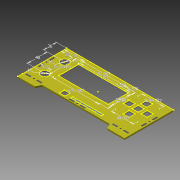
# Autodesk Inventor part: Front Panel
Saved by Autodesk Inventor 2014 (Build 180170000, 170)
## iProperties
Created: 2013-07-14
Part Number: Front Panel
Material: Generic
Document SubType Name: Modeling
Designer: james
Density: 1 g/cm^3
Appearance: Default
Author: james
Autodesk Inventor part; units mm, degrees
ref_plane "YZ Plane" through (0, 0, 0) normal (1, 0, 0) x (0, 1, 0)
ref_plane "XZ Plane" through (0, 0, 0) normal (0, 1, 0) x (-1, 0, 0)
ref_plane "XY Plane" through (0, 0, 0) normal (0, 0, 1) x (1, 0, 0)
sketch "Sketch1" plane through (0, 0, 0) normal (0, 0, 1) x (1, 0, 0)
  line L0 (-107.95, 44.45) -> (107.95, 44.45)
  line L1 (-107.95, -54.45) -> (-72.95, -54.45)
  line L2 (-72.95, -54.45) -> (-67.95, -44.45)
  line L3 (67.95, -44.45) -> (-67.95, -44.45)
  line L4 (107.95, -54.45) -> (72.95, -54.45)
  line L5 (72.95, -54.45) -> (67.95, -44.45)
  line L6 (-107.95, 44.45) -> (-107.95, -54.45)
  line L7 (107.95, 44.45) -> (107.95, -54.45)
  point P0 (0, 0)
  dimension "d36" = 88.9
  dimension "d38" = 215.9
  dimension "d39" = 44.45
  dimension "d40" = 107.95
  dimension "d41" = 98.9
  dimension "d42" = 10
  dimension "d43" = 116.565
  dimension "d44" = 35
  dimension "d45" = 35
  dimension "d46" = 116.565
  dimension "d47" = 40
  constraints: 16 end point, 2 parallel, 1 horizontal, 1 perpendicular
  measures "d36" distance between parallel lines of L3 L0
  measures "d38" distance of L0.start L0.end
  measures "d39" distance from line of point (0, 0) L0
  measures "d40" distance from line of point (0, 0) L6
  measures "d41" distance of L0.start L1.start
  measures "d42" distance between parallel lines of L1 L3
  measures "d43" angle of L1 L2
  measures "d44" distance of L4.start L4.end
  measures "d45" distance of L1.start L1.end
  measures "d46" angle of L4 L5
  measures "d47" distance from line of L7 L3.start
extrude "Face ext" add sketch "Sketch1" along normal blind 3
sketch "Cutouts - skt" plane through (0, 0, 3) normal (0, 0, 1) x (1, 0, 0)
  line L0 (107.95, 44.45) -> (-107.95, 44.45) projected
  line L1 (63.8676, -13.289) -> (63.8676, -1.2663)
  line L2 (75.89, -13.289) -> (63.8676, -13.289)
  line L3 (75.89, -1.2663) -> (75.89, -13.289)
  line L4 (63.8676, -1.2663) -> (75.89, -1.2663)
  line L5 (46.0028, 16.7255) -> (58.0255, 16.7255)
  line L6 (46.0028, 4.7026) -> (46.0028, 16.7255)
  line L7 (58.0255, 4.7026) -> (46.0028, 4.7026)
  line L8 (58.0255, 16.7255) -> (58.0255, 4.7026)
  line L9 (75.9748, 33.8704) -> (75.9748, 21.8478)
  line L10 (63.9944, 33.8704) -> (75.9748, 33.8704)
  line L11 (63.9944, 21.8478) -> (63.9944, 33.8704)
  line L12 (75.9748, 21.8478) -> (63.9944, 21.8478)
  line L13 (63.9521, 16.7677) -> (75.9324, 16.7677)
  line L14 (63.9521, 4.7874) -> (63.9521, 16.7677)
  line L15 (75.9324, 4.7874) -> (63.9521, 4.7874)
  line L16 (75.9324, 16.7677) -> (75.9324, 4.7874)
  line L17 (94.0088, 4.8721) -> (94.0088, 16.8525)
  line L18 (82.0285, 4.8721) -> (94.0088, 4.8721)
  line L19 (82.0285, 16.8525) -> (82.0285, 4.8721)
  line L20 (94.0088, 16.8525) -> (82.0285, 16.8525)
  line L21 (27.7989, -11.6866) -> (-67.95, -11.6866)
  line L22 (-67.95, 28.3134) -> (25.7989, 28.3134)
  line L23 (32.0499, 28.3134) -> (32.0499, -11.6866)
  circle A0 centre (-85.95, 18.45) radius 8
  circle A1 centre (-85.95, -21.55) radius 8
  line L24 (-67.95, 28.3134) -> (32.0499, 28.3134)
  line L25 (32.0499, 28.3134) -> (32.0499, -11.6866)
  line L26 (32.0499, -11.6866) -> (-67.95, -11.6866)
  line L27 (-67.95, -11.6866) -> (-67.95, 28.3134)
  line L28 (63.9944, 33.8704) -> (75.9748, 33.8704)
  line L29 (75.9748, 33.8704) -> (75.9748, 21.8478)
  line L30 (75.9748, 21.8478) -> (63.9944, 21.8478)
  line L31 (63.9944, 21.8478) -> (63.9944, 33.8704)
  line L32 (82.0285, 16.8525) -> (94.0088, 16.8525)
  line L33 (94.0088, 16.8525) -> (94.0088, 4.8721)
  line L34 (94.0088, 4.8721) -> (82.0285, 4.8721)
  line L35 (82.0285, 4.8721) -> (82.0285, 16.8525)
  line L36 (63.9521, 16.7677) -> (75.9324, 16.7677)
  line L37 (75.9324, 16.7677) -> (75.9324, 4.7874)
  line L38 (75.9324, 4.7874) -> (63.9521, 4.7874)
  line L39 (63.9521, 4.7874) -> (63.9521, 16.7677)
  line L40 (46.0028, 16.7255) -> (58.0255, 16.7255)
  line L41 (58.0255, 16.7255) -> (58.0255, 4.7026)
  line L42 (58.0255, 4.7026) -> (46.0028, 4.7026)
  line L43 (46.0028, 4.7026) -> (46.0028, 16.7255)
  line L44 (63.8676, -1.2663) -> (75.89, -1.2663)
  line L45 (75.89, -1.2663) -> (75.89, -13.289)
  line L46 (75.89, -13.289) -> (63.8676, -13.289)
  line L47 (63.8676, -13.289) -> (63.8676, -1.2663)
  line L48 (-36.7815, -30.9654) -> (-26.011, -30.9654)
  line L49 (-26.011, -30.9654) -> (-26.011, -40.9281)
  line L50 (-26.011, -40.9281) -> (-36.7815, -40.9281)
  line L51 (-36.7815, -40.9281) -> (-36.7815, -30.9654)
  line L52 (-16.5867, -34.4658) -> (45.1738, -34.4658) construction
  line L53 (45.1738, -34.4658) -> (45.1738, -38.1955) construction
  line L54 (45.1738, -38.1955) -> (-16.5867, -38.1955) construction
  line L55 (-16.5867, -38.1955) -> (-16.5867, -34.4658) construction
  line L56 (-107.95, 44.45) -> (-107.95, -54.45) projected
  point P0 (-107.95, -44.45)
  point P1 (0, 0)
  point P2 (-70.7327, 35.8725)
  point P3 (22.3305, 35.8725)
  point P4 (22.3305, -19.1888)
  point P5 (-70.7327, -19.1888)
  point P6 (48.035, 31.7962)
  point P7 (92.0616, 31.7962)
  point P8 (48.035, -12.2207)
  point P9 (92.0616, -12.2207)
  point P10 (48.035, 31.7962)
  point P11 (92.0616, 31.7962)
  point P12 (92.0616, -12.2207)
  point P13 (48.035, -12.2207)
  point P14 (-70.7327, 35.8725)
  point P15 (22.3305, 35.8725)
  point P16 (22.3305, -19.1888)
  point P17 (-70.7327, -19.1888)
  dimension "d8" = 16
  dimension "d9" = 16
  dimension "d13" = 26
  dimension "d48" = 40
  dimension "d49" = 99.9999
  dimension "d50" = 40
  dimension "d51" = 93.0632
  dimension "d52" = 93.0632
  dimension "d53" = 55.0612
  dimension "d54" = 55.0612
  dimension "d55" = 8.5775
  dimension "d57" = 7.5591
  dimension "d59" = 44.0266
  dimension "d60" = 44.0266
  dimension "d61" = 22
  dimension "d62" = 22
  dimension "d90" = 40
  dimension "d91" = 18
  constraints: 102 end point, 14 parallel, 8 coincident, 7 horizontal, 7 perpendicular, 2 centre point, 2 other
  measures "d8" diameter of A0
  measures "d9" diameter of A1
  measures "d13" distance from line of L0 A0.centre
  measures "d48" distance of A1.centre A0.centre
  measures "d49" distance of L22.start L24.end
  measures "d50" distance of L23.start L23.end
  measures "d51" distance of point (22.331, 35.872) point (-70.733, 35.872)
  measures "d52" distance of point (22.331, -19.189) point (-70.733, -19.189)
  measures "d53" distance of point (22.331, -19.189) point (22.331, 35.872)
  measures "d54" distance of point (-70.733, -19.189) point (-70.733, 35.872)
  measures "d55" distance from line of L0 point (22.331, 35.872)
  measures "d57" distance from line of L22 point (22.331, 35.872)
  measures "d59" distance of point (92.062, -12.221) point (48.035, -12.221)
  measures "d60" distance of point (92.062, 31.796) point (48.035, 31.796)
  measures "d61" distance from line of L56 A0.centre
  measures "d62" distance from line of L56 A1.centre
  measures "d90" distance between parallel lines of L56 L27
  measures "d91" distance from line of L27 A0.centre
sketch3d "3D Sketch1"
extrude "Cut-outs ext" cut sketch "Cutouts - skt" against normal through all
hole "Hole1" at (-70.7327, 35.8725, 3) at (-70.7327, -19.1888, 3) at (22.3305, -19.1888, 3) at (22.3305, 35.8725, 3) at (48.035, -12.2207, 3) at (48.035, 31.7962, 3) at (92.0616, 31.7962, 3) at (92.0616, -12.2207, 3) direction (0, 0, -1) diameter 3 end through all
sketch "Mating Holes" plane through (0, 0, 3) normal (0, 0, 1) x (1, 0, 0)
  line L0 (107.95, 44.45) -> (-107.95, 44.45) projected
  line L1 (-107.95, 44.45) -> (-107.95, -54.45) projected
  line L2 (-67.95, -44.45) -> (67.95, -44.45) projected
  line L3 (107.95, -54.45) -> (107.95, 44.45) projected
  circle A0 centre (-103.95, 0) radius 1.5
  line L4 (-105.5, -6) -> (-102.4, -6)
  line L5 (-102.4, -6) -> (-102.4, -16.1)
  line L6 (-102.4, -16.1) -> (-105.5, -16.1)
  line L7 (-105.5, -16.1) -> (-105.5, -6)
  line L8 (-105.5, 16.0999) -> (-102.4, 16.0999)
  line L9 (-102.4, 16.0999) -> (-102.4, 5.9999)
  line L10 (-102.4, 5.9999) -> (-105.5, 5.9999)
  line L11 (-105.5, 5.9999) -> (-105.5, 16.0999)
  circle A1 centre (103.95, 0) radius 1.5
  line L12 (102.4, -6) -> (105.5, -6)
  line L13 (105.5, -6) -> (105.5, -16.1)
  line L14 (105.5, -16.1) -> (102.4, -16.1)
  line L15 (102.4, -16.1) -> (102.4, -6)
  line L16 (102.4, 16.0999) -> (105.5, 16.0999)
  line L17 (105.5, 16.0999) -> (105.5, 5.9999)
  line L18 (105.5, 5.9999) -> (102.4, 5.9999)
  line L19 (102.4, 5.9999) -> (102.4, 16.0999)
  point P0 (0, 0)
  dimension "d63" = 3
  dimension "d75" = 44.45
  dimension "d79" = 3.1
  dimension "d80" = 10.1
  dimension "d81" = 6
  dimension "d85" = 3.1
  dimension "d86" = 10.1
  dimension "d87" = 5.9999
  dimension "d88" = 1.55
  dimension "d89" = 1.55
  dimension "d92" = 3
  dimension "d93" = 3.1
  dimension "d94" = 10.1
  dimension "d95" = 6
  dimension "d96" = 3.1
  dimension "d97" = 10.1
  dimension "d98" = 5.9999
  dimension "d99" = 1.55
  dimension "d100" = 1.55
  dimension "d101" = 4
  dimension "d102" = 44.45
  dimension "d103" = 4
  dimension "d104" = 88.9
  constraints: 32 end point, 8 parallel, 4 horizontal, 4 perpendicular, 2 centre point
  measures "d63" diameter of A0
  measures "d75" distance from line of L0 A0.centre
  measures "d79" distance of L5.end L6.end
  measures "d80" distance of L4.end L5.end
  measures "d81" vertical distance of L4.end A0.centre
  measures "d85" distance of L9.end L10.end
  measures "d86" distance of L8.end L9.end
  measures "d87" distance from line of L10 A0.centre
  measures "d88" distance from line of A0.centre L9
  measures "d89" distance from line of L5 A0.centre
  measures "d92" diameter of A1
  measures "d93" distance of L14.start L14.end
  measures "d94" distance of L13.start L14.start
  measures "d95" vertical distance of L13.start A1.centre
  measures "d96" distance of L18.start L18.end
  measures "d97" distance of L17.start L18.start
  measures "d98" distance from line of L18 A1.centre
  measures "d99" distance from line of A1.centre L17
  measures "d100" distance from line of L13 A1.centre
  measures "d101" distance from line of L3 A1.centre
  measures "d102" distance from line of L0 A1.centre
  measures "d103" distance from line of L1 A0.centre
  measures "d104" distance between parallel lines of L2 L0
extrude "Side Panel Slots" cut sketch "Mating Holes" against normal through all
sketch "Bottom Panel Slots" plane through (0, 0, 3) normal (0, 0, 1) x (1, 0, 0)
  line L0 (-107.95, 44.45) -> (-107.95, -54.45) projected
  line L1 (-107.95, -54.45) -> (-72.95, -54.45) projected
  line L2 (72.95, -54.45) -> (107.95, -54.45) projected
  circle A0 centre (-87.945, -41.45) radius 1.5
  line L3 (-93.945, -39.9) -> (-104.045, -39.9)
  line L4 (-104.045, -39.9) -> (-104.045, -43)
  line L5 (-104.045, -43) -> (-93.945, -43)
  line L6 (-93.945, -43) -> (-93.945, -39.9)
  line L7 (-81.945, -39.9) -> (-71.845, -39.9)
  line L8 (-71.845, -39.9) -> (-71.845, -43)
  line L9 (-71.845, -43) -> (-81.945, -43)
  line L10 (-81.945, -43) -> (-81.945, -39.9)
  circle A1 centre (87.013, -41.45) radius 1.5
  line L11 (93.013, -42.95) -> (103.113, -42.95)
  line L12 (103.113, -42.95) -> (103.113, -39.85)
  line L13 (103.113, -39.85) -> (93.013, -39.85)
  line L14 (93.013, -39.85) -> (93.013, -42.95)
  line L15 (81.013, -39.85) -> (70.913, -39.85)
  line L16 (70.913, -39.85) -> (70.913, -42.95)
  line L17 (70.913, -42.95) -> (81.013, -42.95)
  line L18 (81.013, -42.95) -> (81.013, -39.85)
  circle A2 centre (-0.45, -41.45) radius 1.5
  line L19 (5.55, -42.95) -> (15.65, -42.95)
  line L20 (15.65, -42.95) -> (15.65, -39.85)
  line L21 (15.65, -39.85) -> (5.55, -39.85)
  line L22 (5.55, -39.85) -> (5.55, -42.95)
  line L23 (-6.45, -39.85) -> (-16.55, -39.85)
  line L24 (-16.55, -39.85) -> (-16.55, -42.95)
  line L25 (-16.55, -42.95) -> (-6.45, -42.95)
  line L26 (-6.45, -42.95) -> (-6.45, -39.85)
  point P0 (0, 0)
  point P1 (-93.945, -41.45)
  point P2 (-71.845, -41.45)
  dimension "d109" = 3
  dimension "d112" = 10.1
  dimension "d113" = 3.1
  dimension "d116" = 13
  dimension "d118" = 10.1
  dimension "d119" = 3.1
  dimension "d120" = 13
  dimension "d123" = 6
  dimension "d124" = 6
  dimension "d125" = 13
  dimension "d129" = 3
  dimension "d130" = 10.1
  dimension "d131" = 3.1
  dimension "d132" = 10.1
  dimension "d133" = 3.1
  dimension "d134" = 6
  dimension "d137" = 6
  dimension "d138" = 13
  dimension "d140" = 1.5
  dimension "d141" = 1.5
  dimension "d142" = 3
  dimension "d143" = 107.5
  dimension "d144" = 13
  dimension "d145" = 10.1
  dimension "d146" = 3.1
  dimension "d147" = 10.1
  dimension "d148" = 3.1
  dimension "d149" = 1.5
  dimension "d150" = 1.5
  dimension "d151" = 6
  dimension "d152" = 6
  dimension "d155" = 87.463
  dimension "d156" = 87.495
  constraints: 48 end point, 12 parallel, 6 horizontal, 6 perpendicular, 3 centre point, 2 midpoint
  measures "d109" diameter of A0
  measures "d112" distance of L5.end L4.end
  measures "d113" distance of L4.end L3.end
  measures "d116" distance from line of L1 point (-93.945, -41.45)
  measures "d118" distance of L8.end L9.end
  measures "d119" distance of L7.end L8.end
  measures "d120" distance from line of L1 point (-71.845, -41.45)
  measures "d123" distance from line of A0.centre L6
  measures "d124" distance from line of L10 A0.centre
  measures "d125" distance from line of L1 A0.centre
  measures "d129" diameter of A1
  measures "d130" distance of L13.end L12.end
  measures "d131" distance of L12.end L11.end
  measures "d132" distance of L17.end L16.end
  measures "d133" distance of L16.end L15.end
  measures "d134" distance from line of L14 A1.centre
  measures "d137" distance from line of L18 A1.centre
  measures "d138" distance from line of L2 A1.centre
  measures "d140" distance from line of A1.centre L11
  measures "d141" distance from line of L17 A1.centre
  measures "d142" diameter of A2
  measures "d143" distance from line of L0 A2.centre
  measures "d144" distance from line of L1 A2.centre
  measures "d145" distance of L21.end L20.end
  measures "d146" distance of L20.end L19.end
  measures "d147" distance of L25.end L24.end
  measures "d148" distance of L24.end L23.end
  measures "d149" distance from line of L25 A2.centre
  measures "d150" distance from line of A2.centre L19
  measures "d151" distance from line of L26 A2.centre
  measures "d152" distance from line of L22 A2.centre
  measures "d155" distance of A1.centre A2.centre
  measures "d156" distance of A2.centre A0.centre
extrude "Extrusion4" cut sketch "Bottom Panel Slots" against normal blind 10
equation "\"d39\" = 0.5 * d36"
equation "\"d40\" = 0.5 * d38"
equation "\"d45\" = d44"
equation "\"d46\" = d43"
equation "\"d52\" = d51"
equation "\"d54\" = d53"
equation "\"d60\" = d59"
equation "\"d62\" = d61"
equation "\"d75\" = 0.5 * d104"
equation "\"d79\" = d85"
equation "\"d80\" = d86"
equation "\"d88\" = 0.5 * d85"
equation "\"d89\" = d88"
equation "\"d93\" = d96"
equation "\"d94\" = d97"
equation "\"d99\" = 0.5 * d96"
equation "\"d100\" = d99"
equation "\"d101\" = d84"
equation "\"d102\" = d75"
equation "\"d105\" = d76"
equation "\"d84\" = 4"
equation "\"d76\" = 88.9"
body "Solid1"
